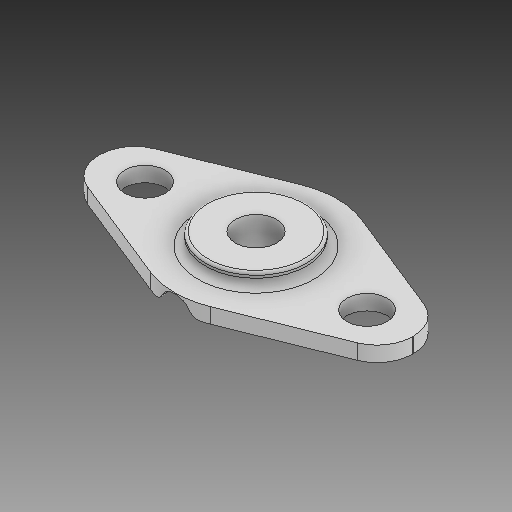
# Autodesk Inventor part: HD_rotor
Saved by Autodesk Inventor 2020 (Build 240168000, 168)
## iProperties
Created: 2021-03-19
Part Number: HD_rotor
Material: Generic
Document SubType Name: Modeling
Designer: DDeGo
Density: 1 g/cm^3
Appearance: Default
Author: DDeGo
Autodesk Inventor part; units mm, degrees
ref_plane "YZ Plane" through (0, 0, 0) normal (1, 0, 0) x (0, 1, 0)
ref_plane "XZ Plane" through (0, 0, 0) normal (0, 1, 0) x (-1, 0, 0)
ref_plane "XY Plane" through (0, 0, 0) normal (0, 0, 1) x (1, 0, 0)
sketch "608 bearing" plane through (0, 0, 0) normal (0, 0, 1) x (1, 0, 0)
  line L0 (-83.9037, 39.6189) -> (-76.9037, 39.6189) construction
  line L1 (-61.9037, 39.6189) -> (-61.9037, 32.6189) construction
  line L2 (-61.9037, 32.6189) -> (-68.9037, 32.6189) construction
  line L3 (-83.9037, 32.6189) -> (-83.9037, 39.6189) construction
  line L4 (-76.9037, 39.6189) -> (-76.9037, 32.6189) construction
  line L5 (-68.9037, 39.6189) -> (-68.9037, 32.6189) construction
  line L6 (-68.9037, 39.6189) -> (-61.9037, 39.6189) construction
  line L7 (-76.9037, 39.6189) -> (-68.9037, 39.6189) construction
  line L8 (-76.9037, 32.6189) -> (-83.9037, 32.6189) construction
  line L9 (-68.9037, 32.6189) -> (-76.9037, 32.6189) construction
  point P0 (-72.9037, 36.1189)
  point P1 (-72.9037, 39.6189)
  point P2 (-72.9037, 32.6189)
  dimension "d24" = 7
  dimension "d25" = 22
  dimension "d26" = 8
  measures "d24" distance of L1.start L1.end
  measures "d25" distance between parallel lines of L1 L3
  measures "d26" distance between parallel lines of L5 L4
derived "HD_mastersketch.ipt"
sketch "Belt" plane through (0, 0, 0) normal (0, 0, 1) x (1, 0, 0)
  line L0 (-33.9, 7.5) -> (-33.1, 7.5)
  line L1 (-33.1, 7.5) -> (-33.1, -7.5)
  line L2 (-33.1, -7.5) -> (-33.9, -7.5)
  line L3 (-33.9, -7.5) -> (-33.9, 7.5)
  point P0 (0, 0)
  point P1 (-33.9, 0)
sketch "Rotor" plane through (0, 0, 0) normal (0, 0, 1) x (1, 0, 0)
  line L0 (0, 0) -> (0, -29.5)
  line L1 (0, -29.5) -> (-4.075, -29.5)
  line L2 (-4.075, -29.5) -> (-4.075, -4.5)
  line L3 (-11.5, -1.5) -> (-31.1, -1.5)
  line L4 (-31.1, -1.5) -> (-31.1, 1.5)
  line L5 (-31.1, 1.5) -> (-11.5, 1.5)
  line L6 (-4.075, 1.5) -> (-4.075, -4.5)
  line L7 (-4.075, 1.5) -> (-4.075, 13.5)
  line L8 (-4.075, 13.5) -> (0, 13.5)
  line L9 (0, 13.5) -> (0, 0)
  line L10 (-33.1, 7.5) -> (-33.1, -7.5) construction
  line L11 (-33.1, 0) -> (-31.1, 0) construction
  line L12 (-22, -2) -> (-22, -1.5) construction
  line L13 (-22, -1.5) -> (-22, 1.5) construction
  line L14 (-22, 2) -> (-22, 1.5) construction
  line L15 (-26.05, 1.5) -> (-26.05, -1.5) construction
  line L16 (-17.95, -1.5) -> (-17.95, 1.5) construction
  line L17 (-9.5, 1.5) -> (-9.5, -1.5) construction
  line L18 (-9.5, -3.5) -> (-9.5, -4)
  line L19 (-9, -4.5) -> (-4.075, -4.5)
  line L20 (-9.5, 1.5) -> (-9.5, 1.5)
  line L21 (-9.5, 1.5) -> (-9.5, -4.5) construction
  line L22 (-9.5, 1.5) -> (-4.075, 1.5)
  line L23 (-26.05, 0) -> (-22, 0) construction
  line L24 (-22, 0) -> (-17.95, 0) construction
  arc A0 (-9.5, -3.5) -> (-11.5, -1.5) centre (-11.5, -3.5) ccw
  arc A1 (-9.5, -4) -> (-9, -4.5) centre (-9, -4) ccw
  arc A2 (-11.5, 1.5) -> (-10, 3) centre (-11.5, 3) ccw
  arc A3 (-9.5, 4) -> (-10, 3.5) centre (-9.5, 3.5) ccw
  line L25 (-10, 3) -> (-10, 3.5)
  line L26 (-11.5, -1.5) -> (-11.5, 1.5) construction
  line L27 (-9.5, 4) -> (-4.075, 4)
  line L28 (-11.5, 1.5) -> (-9.5, 1.5) construction
  line L29 (-33, 9) -> (-26, 9) construction
  line L30 (-11, 9) -> (-11, 2) construction
  line L31 (-11, 2) -> (-18, 2) construction
  line L32 (-33, 2) -> (-33, 9) construction
  line L33 (-26, 9) -> (-26, 2) construction
  line L34 (-18, 9) -> (-18, 2) construction
  line L35 (-18, 9) -> (-11, 9) construction
  line L36 (-26, 9) -> (-18, 9) construction
  line L37 (-26, 2) -> (-33, 2) construction
  line L38 (-18, 2) -> (-26, 2) construction
  line L39 (-33, -2) -> (-26, -2) construction
  line L40 (-11, -2) -> (-11, -9) construction
  line L41 (-11, -9) -> (-18, -9) construction
  line L42 (-33, -9) -> (-33, -2) construction
  line L43 (-26, -2) -> (-26, -9) construction
  line L44 (-18, -2) -> (-18, -9) construction
  line L45 (-18, -2) -> (-11, -2) construction
  line L46 (-26, -2) -> (-18, -2) construction
  line L47 (-26, -9) -> (-33, -9) construction
  line L48 (-18, -9) -> (-26, -9) construction
  point P0 (-9.35, 1.5)
sketch "Base" plane through (0, 0, 0) normal (0, 0, 1) x (1, 0, 0)
  line L0 (0, -14.2) -> (-8.1, -14.2) construction
  line L1 (-40, -13.2) -> (-40, -1.25)
  line L2 (-39, -0.25) -> (-34, -0.25)
  line L3 (-28, -11.5) -> (-16, -11.5)
  line L4 (-10.5, -10) -> (-9.1, -6.2)
  line L5 (-9.1, -6.2) -> (-7.1, -6.2)
  line L6 (-7.1, -6.2) -> (-7.1, -7.7)
  line L7 (-7.1, -7.7) -> (-8.1, -8.7)
  line L8 (-8.1, -8.7) -> (-8.1, -14.2)
  line L9 (-8.1, -14.2) -> (-39, -14.2)
  line L10 (0, -14.2) -> (0, 38.4357) construction
  line L11 (-34, -0.25) -> (-34, -8)
  line L12 (-34, -8) -> (-32.5, -10)
  line L13 (-28, -10) -> (-28, -11.5)
  line L14 (-39, -0.25) -> (-40, -1.25)
  line L15 (-40, -13.2) -> (-39, -14.2)
  line L16 (-16, -11.5) -> (-16, -10)
  line L17 (-16, -10) -> (-10.5, -10)
  line L18 (-32.5, -10) -> (-28, -10)
  line L19 (0, 0) -> (-64.9444, 0) construction
  line L20 (-16, 11.5) -> (-16, 10)
  line L21 (-16, 10) -> (-10.5, 10)
  line L22 (-10.5, 10) -> (-9.1, 5.5)
  line L23 (-9.1, 5.5) -> (-7.1, 5.5)
  line L24 (-8.1, 8) -> (-8.1, 13.5)
  line L25 (-7.1, 5.5) -> (-7.1, 7)
  line L26 (-7.1, 7) -> (-8.1, 8)
  line L27 (0.103, 13.5) -> (-8.1, 13.5) construction
  line L28 (-28, 11.5) -> (-16, 11.5)
  line L29 (-8.1, 13.5) -> (-36.45, 13.5)
  line L30 (-37.45, 12.5) -> (-37.45, 2.8)
  line L31 (-38.25, 0.25) -> (-34, 0.25)
  line L32 (-28, 10) -> (-28, 11.5)
  line L33 (-32.5, 10) -> (-28, 10)
  line L34 (-34, 8) -> (-32.5, 10)
  line L35 (-34, 0.25) -> (-34, 8)
  line L36 (-37.45, 12.5) -> (-36.45, 13.5)
  line L37 (-38.25, 2) -> (-37.45, 2.8)
  line L38 (-33.9, -7.5) -> (-33.9, 7.5) construction
  line L39 (-33.1, -7.5) -> (-33.9, -7.5) construction
  line L40 (-22, -9) -> (-22, -11.5) construction
  line L41 (-30, 13.5) -> (-30, 12) construction
  line L42 (-30, 12) -> (-30, 10) construction
  line L43 (-30, -14.2) -> (-30, -12) construction
  line L44 (-26, -9) -> (-33, -9) construction
  line L45 (-9.5, -4.5) -> (-4.075, -4.5)
  line L46 (-9.5, 1.5) -> (-4.075, 1.5)
  line L47 (-8.1, 8) -> (-8.1, -8.7) construction
  line L48 (-38.25, 2) -> (-38.25, 0.25)
  line L49 (-30, -12) -> (-30, -10) construction
  point P0 (-40, -14.2)
  point P1 (-40, -0.25)
  point P2 (-37.45, 13.5)
  point P3 (-37.45, 0.25)
  point P4 (-22, 11.5)
revolve "Revolution1" add sketch "Rotor" angle 360 about axis through (0, 13.5, 0) along (0, -1, 0) contours L19 A1 L18 A0 L3 L4 L5 A2 L25 A3 L27 L7 L6
sketch "Sketch8" plane through (0, 1.5, 0) normal (0, 1, 0) x (1, 0, 0)
  circle A0 centre (0, 0) radius 31.1 projected
  line L0 (-30.6954, -5) -> (-6.0117, -14.9355)
  line L1 (-30.6954, -5) -> (-30.6954, 5) construction
  line L2 (-30.6954, 5) -> (-6.0117, 14.9355)
  circle A1 centre (0, 0) radius 4 construction
  line L3 (6.0117, -14.9355) -> (30.6954, -5)
  line L4 (30.6954, -5) -> (30.6954, 5) construction
  line L5 (30.6954, 5) -> (6.0117, 14.9355)
  arc A2 (-6.0117, -14.9355) -> (6.0117, -14.9355) centre (0, 0) ccw
  arc A3 (6.0117, 14.9355) -> (-6.0117, 14.9355) centre (0, 0) ccw
  point P0 (0, 0)
  dimension "d4" = 10
  dimension "d5" = 15
  constraints: 12 end point, 8 point on circle, 3 equal length, 2 centre point, 2 tangent, 2 vertical, 1 coincident, 1 concentric
  measures "d4" distance of L0.start L1.end
  measures "d5" radial gap between concentric circles of A0 A2
extrude "Extrusion1" cut sketch "Sketch8" against normal through all contours L5 A3 L2 A0 | A0 L0 A2 L3
sketch "Sketch9" plane through (0, 1.5, 0) normal (0, 1, 0) x (1, 0, 0)
  circle A0 centre (-22, 0) radius 4
  circle A1 centre (22, 0) radius 4
  circle A2 centre (0, 0) radius 16.1459 projected
  circle A3 centre (0, 0) radius 4.075 projected
  line L0 (0, 0) -> (0, 28.0271) construction
  point P0 (-26, 0)
  constraints: 2 end point, 1 centre point, 1 coincident, 1 horizontal alignment, 1 vertical, 3 other
extrude "Extrusion2" cut sketch "Sketch9" against normal through all contours A0 | A1
fillet "Fillet1" radius 7 4 edges at (30.6954, 0, 5) (30.6954, 0, -5) (-30.6954, 0, -5) (-30.6954, 0, 5)
sketch "Sketch10" plane through (0, -4.5, 0) normal (0, 1, 0) x (1, 0, 0)
  line L0 (-2.85, -5.9) -> (2.85, -5.9)
  line L1 (2.85, -5.9) -> (2.85, -3.6)
  line L2 (2.85, -3.6) -> (-2.85, -3.6)
  line L3 (-2.85, -3.6) -> (-2.85, -5.9)
  line L4 (-2.85, -5.9) -> (2.85, -3.6) construction
  line L5 (2.85, -5.9) -> (-2.85, -3.6) construction
  line L6 (0, 0) -> (0, -4.75) construction
  dimension "d11" = 3.6
  dimension "d12" = 2.3
  dimension "d13" = 5.7
  constraints: 14 end point, 2 midpoint, 2 parallel, 1 horizontal, 1 perpendicular, 1 vertical
  measures "d11" distance from line of L6.start L2
  measures "d12" distance of L0.end L1.end
  measures "d13" distance of L0.start L0.end
extrude "Extrusion3" cut sketch "Sketch10" along normal blind 5.7
sketch "Sketch14" plane through (0, 0, 0) normal (1, 0, 0) x (0, 1, 0)
  line L0 (-1.65, 5.9) -> (-1.65, 28.5259)
  line L1 (-1.65, 5.9) -> (0, 5.9)
  line L2 (0, 5.9) -> (0, 9.9)
  line L3 (0, 9.9) -> (1.35, 9.9)
  line L4 (1.35, 9.9) -> (1.35, 19.9)
  line L5 (1.35, 19.9) -> (-0.15, 19.9)
  line L6 (-0.15, 19.9) -> (-0.15, 28.5259)
  line L7 (-0.15, 28.5259) -> (-1.65, 28.5259)
  line L8 (-4.5, 5.9) -> (1.2, 5.9) projected
  point P0 (0, 0)
  point P1 (1.5, 0)
  point P2 (1.2, 5.9)
  point P3 (-3.604, 6.2)
  dimension "d29" = 1.65
  dimension "d30" = 3
  dimension "d32" = 10
  dimension "d33" = 1.5
  dimension "d36" = 4
  constraints: 16 end point, 5 perpendicular, 2 vertical, 1 horizontal, 2 other
  measures "d29" distance between parallel lines of L0 L2
  measures "d30" distance between parallel lines of L0 L4
  measures "d32" distance of L3.end L4.end
  measures "d33" distance between parallel lines of L0 L6
revolve "Revolution2" cut sketch "Sketch14" angle 360 about axis through (0, -1.65, 5.9) along (0, 0, 1)
fillet "Fillet3" radius 2 2 edges at (2.9994, -1.5906, 10.4842) (-2.9994, -1.5906, 10.4842)
body "Solid1"
